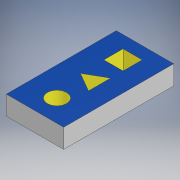
# Autodesk Inventor part: Pegboard new
Saved by Autodesk Inventor 2018 (Build 220112000, 112)
## iProperties
Created: 2021-02-05
Part Number: Pegboard new
Material: Generic
Document SubType Name: Modeling
Designer: Bell539x
Density: 1 g/cm^3
Appearance: Default
Author: Bell539x
Autodesk Inventor part; units mm, degrees
ref_plane "YZ Plane" through (0, 0, 0) normal (1, 0, 0) x (0, 1, 0)
ref_plane "XZ Plane" through (0, 0, 0) normal (0, 1, 0) x (-1, 0, 0)
ref_plane "XY Plane" through (0, 0, 0) normal (0, 0, 1) x (1, 0, 0)
sketch "Sketch1" plane through (0, 0, 0) normal (0, 1, 0) x (-1, 0, 0)
  line L0 (49.6769, 99.8505) -> (-26.5231, 99.8505)
  line L1 (-26.5231, 99.8505) -> (-26.5231, -46.1995)
  line L2 (-26.5231, -46.1995) -> (49.6769, -46.1995)
  line L3 (49.6769, -46.1995) -> (49.6769, 99.8505)
  point P0 (0, 0)
  dimension "d0" = 146.05
  dimension "d1" = 76.2
  constraints: 8 end point, 2 parallel, 1 horizontal, 1 perpendicular
  measures "d0" distance of L2.end L0.start
  measures "d1" distance of L1.end L2.end
extrude "Extrusion1" add sketch "Sketch1" along normal blind 25.4
sketch "Sketch2" plane through (0, 25.4, 0) normal (0, 1, 0) x (1, 0, 0)
  circle A0 centre (-11.5769, -70.6659) radius 12.7
  line L0 (-49.6769, 46.1995) -> (-49.6769, -99.8505) projected
  line L1 (-49.6769, -99.8505) -> (26.5231, -99.8505) projected
  point P0 (0, 0)
  dimension "d4" = 25.4
  dimension "d5" = 38.1
  dimension "d6" = 29.1846
  constraints: 1 centre point
  measures "d4" diameter of A0
  measures "d5" distance from line of A0.centre L0
  measures "d6" distance from line of A0.centre L1
extrude "Extrusion2" cut sketch "Sketch2" against normal blind 25.4
sketch "Sketch3" plane through (0, 25.4, 0) normal (0, 1, 0) x (1, 0, 0)
  line L0 (-24.2769, 4.3149) -> (1.1231, 4.3149)
  line L1 (1.1231, 4.3149) -> (1.1231, 29.7149)
  line L2 (1.1231, 29.7149) -> (-24.2769, 29.7149)
  line L3 (-24.2769, 29.7149) -> (-24.2769, 4.3149)
  line L4 (26.5231, 46.1995) -> (-49.6769, 46.1995) projected
  line L5 (26.5231, -99.8505) -> (26.5231, 46.1995) projected
  point P0 (0, 0)
  dimension "d9" = 25.4
  dimension "d10" = 16.4846
  dimension "d11" = 25.4
  constraints: 8 end point, 2 parallel, 2 perpendicular, 1 horizontal
  measures "d9" distance of L2.end L0.start
  measures "d10" distance between parallel lines of L4 L2
  measures "d11" distance between parallel lines of L5 L1
extrude "Extrusion3" cut sketch "Sketch3" against normal blind 25.4
sketch "Sketch4" plane through (0, 25.4, 0) normal (0, 1, 0) x (1, 0, 0)
  line L0 (1.1231, -12.1697) -> (1.1231, -41.4813)
  line L1 (1.1231, -41.4813) -> (-24.2769, -26.7988)
  line L2 (-24.2769, -26.7988) -> (1.1231, -12.1697)
  line L3 (26.5231, 46.1995) -> (-49.6769, 46.1995) projected
  line L4 (26.5231, -99.8505) -> (26.5231, 46.1995) projected
  point P0 (0, 0)
  dimension "d14" = 25.4
  dimension "d15" = 29.3116
  dimension "d16" = 58.3692
  dimension "d17" = 25.4
  constraints: 6 end point, 1 equal length, 1 vertical
  measures "d14" horizontal distance of L1.end L0.start
  measures "d15" distance of L0.start L0.end
  measures "d16" distance from line of L0.start L3
  measures "d17" distance between parallel lines of L4 L0
extrude "Extrusion4" cut sketch "Sketch4" against normal blind 25.4
body "Solid1"
